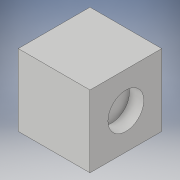
# Autodesk Inventor part: cubo_calibracion_1cm
Saved by Autodesk Inventor 2019 (Build 230136000, 136)
## iProperties
Created: 2019-01-06
Part Number: cubo_calibracion_1cm
Material: Generic
Document SubType Name: Modeling
Designer: assman
Density: 1 g/cm^3
Appearance: Default
Author: assman
## iProperties of the stored document cubo_calibracion_1cm_3DPrint.ipt
Created: 2019-01-06
Part Number: cubo_calibracion_1cm_3DPrint
Material: Generic
Document SubType Name: Modeling
Designer: assman
Density: 1 g/cm^3
Appearance: Default
Author: assman
Autodesk Inventor part; units mm, degrees
ref_plane "YZ Plane" through (0, 0, 0) normal (1, 0, 0) x (0, 1, 0)
ref_plane "XZ Plane" through (0, 0, 0) normal (0, 1, 0) x (-1, 0, 0)
ref_plane "XY Plane" through (0, 0, 0) normal (0, 0, 1) x (1, 0, 0)
sketch "Sketch1" plane through (0, 0, 0) normal (0, 1, 0) x (-1, 0, 0)
  line L0 (5, 5) -> (-5, 5)
  line L1 (-5, 5) -> (-5, -5)
  line L2 (-5, -5) -> (5, -5)
  line L3 (5, -5) -> (5, 5)
  point P0 (0, 0)
  dimension "d0" = 10
  dimension "d1" = 10
  constraints: 8 end point, 2 parallel, 1 horizontal, 1 perpendicular
  measures "d0" distance of L2.end L1.end
  measures "d1" distance of L1.end L0.end
extrude "Extrusion1" add sketch "Sketch1" along normal blind 10
sketch "Sketch2" plane through (5, 0, 5) normal (1, 0, 0) x (0, 0, -1)
  line L0 (0, 0) -> (10, 0) construction
  line L1 (10, 0) -> (10, 10) construction
  line L2 (0, 10) -> (10, 10) construction
  line L3 (0, 0) -> (0, 10) construction
  line L4 (0, 10) -> (10, 10) construction
  line L5 (5, 10) -> (5, 0) construction
  line L6 (0, 0) -> (0, 10) construction
  line L7 (0, 5) -> (10, 5) construction
  line L8 (10, 0) -> (10, 10) construction
  circle A0 centre (5, 5) radius 2.5
  dimension "d4" = 5
  constraints: 4 end point, 4 midpoint, 1 centre point, 1 vertical
  measures "d4" diameter of A0
extrude "Extrusion2" cut sketch "Sketch2" against normal blind 2
body "Solid1"
